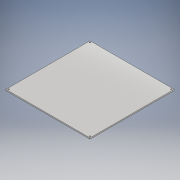
# Autodesk Inventor part: Heated Build Plate
Saved by Autodesk Inventor 2017 (Build 210142000, 142)
## iProperties
Created: 2017-04-02
Part Number: Heated Build Plate
Material: Generic
Document SubType Name: Modeling
Designer: gilef
Density: 1 g/cm^3
Appearance: Aluminum - Polished
Author: gilef
Autodesk Inventor part; units mm, degrees
ref_plane "YZ Plane" through (0, 0, 0) normal (1, 0, 0) x (0, 1, 0)
ref_plane "XZ Plane" through (0, 0, 0) normal (0, 1, 0) x (-1, 0, 0)
ref_plane "XY Plane" through (0, 0, 0) normal (0, 0, 1) x (1, 0, 0)
sketch "Sketch1" plane through (0, 0, 0) normal (0, 0, 1) x (1, 0, 0)
  line L0 (-106.5, -106.5) -> (106.5, -106.5)
  line L1 (106.5, -106.5) -> (106.5, 106.5)
  line L2 (106.5, 106.5) -> (-106.5, 106.5)
  line L3 (-106.5, 106.5) -> (-106.5, -106.5)
  line L4 (-106.5, -106.5) -> (106.5, 106.5) construction
  line L5 (106.5, -106.5) -> (-106.5, 106.5) construction
  point P0 (0, 0)
  dimension "d0" = 213
  constraints: 12 end point, 2 midpoint, 2 parallel, 2 perpendicular, 1 horizontal
  measures "d0" distance of L1.end L2.end
extrude "Extrusion1" add sketch "Sketch1" along normal blind 3
sketch "Sketch2" plane through (0, 0, 3) normal (0, 0, 1) x (1, 0, 0)
  line L0 (-106.5, -106.5) -> (106.5, -106.5) projected
  line L1 (106.5, -106.5) -> (106.5, 106.5) projected
  line L2 (106.5, 106.5) -> (-106.5, 106.5) projected
  line L3 (-106.5, 106.5) -> (-106.5, -106.5) projected
  circle A0 centre (-103, 103) radius 1.5
  line L4 (106.5, 106.5) -> (-106.5, 106.5) construction
  line L5 (0, 106.5) -> (0, -106.5) construction
  line L6 (-106.5, -106.5) -> (106.5, -106.5) construction
  line L7 (-106.5, 0) -> (106.5, 0) construction
  circle A1 centre (103, 103) radius 1.5
  circle A2 centre (-103, -103) radius 1.5
  circle A3 centre (103, -103) radius 1.5
  point P0 (0, 0)
  dimension "d3" = 3
  dimension "d4" = 2
  dimension "d5" = 2
  constraints: 4 centre point, 4 end point, 4 midpoint, 3 symmetric about line, 3 other
  measures "d3" diameter of A0
  measures "d4" distance edge to line of A0 L3
  measures "d5" distance edge to line of A0 L2
extrude "Extrusion2" cut sketch "Sketch2" against normal through all contours A0 | A1 | A2 | A3
body "Solid1"
